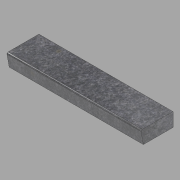
# Autodesk Inventor part: G
Saved by Autodesk Inventor 2022.1 (Build 261234020, 234B)
## iProperties
Created: 2021-12-15
Part Number: G
Material: Granite, Cut, Polished
Document SubType Name: Modeling
Designer: awelt
Density: 2.7 g/cm^3
Appearance: Kasota SN sapphire
Author: awelt
Autodesk Inventor part; units mm, degrees
ref_plane "YZ Plane" through (0, 0, 0) normal (1, 0, 0) x (0, 1, 0)
ref_plane "XZ Plane" through (0, 0, 0) normal (0, 1, 0) x (-1, 0, 0)
ref_plane "XY Plane" through (0, 0, 0) normal (0, 0, 1) x (1, 0, 0)
sketch "Profile" plane through (0, 0, 0) normal (0, 0, 1) x (1, 0, 0)
  line L0 (0, 0) -> (0, 330.2)
  line L1 (0, 0) -> (152.4, 0)
  line L2 (152.4, 0) -> (152.4, 342.9)
  line L3 (152.4, 342.9) -> (139.7, 342.9) construction
  line L4 (152.4, 342.9) -> (139.7, 342.9) construction
  arc A0 (152.4, 342.9) -> (137.4098, 355.3918) centre (139.7, 342.9) ccw
  line L5 (0, 330.2) -> (137.4098, 355.3918)
  dimension "d0" = 330.2
  dimension "d1" = 152.4
  dimension "d2" = 342.9
  dimension "d3" = 12.7
  dimension "d4" = 12.7
  measures "d0" distance of L0.start L0.end
  measures "d1" distance of L0.start L1.end
  measures "d2" distance of L1.end L2.end
  measures "d3" distance of L2.end L3.end
  measures "d4" radius of A0
sketch "Sketch1" plane through (0, 0, 0) normal (1, 0, 0) x (0, 1, 0)
  line L0 (0, 0) -> (0, 330.2)
  line L1 (0, 0) -> (152.4, 0)
  line L2 (152.4, 0) -> (152.4, 342.9)
  line L3 (152.4, 342.9) -> (139.7, 342.9) construction
  line L4 (152.4, 342.9) -> (139.7, 342.9) construction
  arc A0 (152.4, 342.9) -> (137.4098, 355.3918) centre (139.7, 342.9) ccw
  line L5 (0, 330.2) -> (137.4098, 355.3918)
  constraints: 1 other
extrude "Extrusion1" add sketch "Sketch1" along normal blind 1492.25
body "Solid1"
